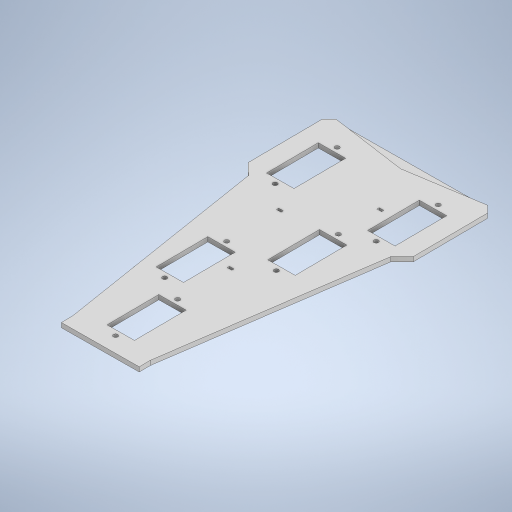
# Autodesk Inventor part: RevisedServoTray
Saved by Autodesk Inventor 2023 (Build 270158000, 158)
## iProperties
Created: 2023-05-02
Part Number: RevisedServoTray
Material: Generic
Document SubType Name: Modeling
Designer: 1roweste
Density: 1 g/cm^3
Appearance: Default
Author: 1roweste
Autodesk Inventor part; units mm, degrees
ref_plane "YZ Plane" through (0, 0, 0) normal (1, 0, 0) x (0, 1, 0)
ref_plane "XZ Plane" through (0, 0, 0) normal (0, 1, 0) x (-1, 0, 0)
ref_plane "Work Plane1" through (0, 2, 0) normal (0, 1, 0) x (1, 0, 0)
sketch "Sketch4" plane through (0, 2, 0) normal (0, 1, 0) x (1, 0, 0)
  line L0 (-81.9697, 60.7) -> (-81.9697, 62.7) projected
  line L1 (-81.9697, 62.7) -> (-80.9697, 62.7) projected
  line L2 (-80.9697, 62.7) -> (-80.9697, 60.7) projected
  line L3 (-80.9697, 60.7) -> (-81.9697, 60.7) projected
  line L4 (-81.9697, 49.6253) -> (-81.9697, 51.6253) projected
  line L5 (-81.9697, 51.6253) -> (-80.9697, 51.6253) projected
  line L6 (-80.9697, 51.6253) -> (-80.9697, 49.6253) projected
  line L7 (-80.9697, 49.6253) -> (-81.9697, 49.6253) projected
  line L8 (-81.9697, 71.7747) -> (-81.9697, 73.7747) projected
  line L9 (-81.9697, 73.7747) -> (-80.9697, 73.7747) projected
  line L10 (-80.9697, 73.7747) -> (-80.9697, 71.7747) projected
  line L11 (-80.9697, 71.7747) -> (-81.9697, 71.7747) projected
  line L12 (-81.9697, 38.5507) -> (-81.9697, 40.5507) projected
  line L13 (-81.9697, 40.5507) -> (-80.9697, 40.5507) projected
  line L14 (-80.9697, 40.5507) -> (-80.9697, 38.5507) projected
  line L15 (-80.9697, 38.5507) -> (-81.9697, 38.5507) projected
  line L16 (-81.9697, 82.8493) -> (-81.9697, 84.8493) projected
  line L17 (-81.9697, 84.8493) -> (-80.9697, 84.8493) projected
  line L18 (-80.9697, 84.8493) -> (-80.9697, 82.8493) projected
  line L19 (-80.9697, 82.8493) -> (-81.9697, 82.8493) projected
  line L20 (-61.9934, 117.9) -> (-84.9697, 94.9237) projected
  line L21 (-84.9697, 94.9237) -> (-89.9697, 61.7) projected
  line L22 (-89.9697, 61.7) -> (-84.9697, 28.4763) projected
  line L23 (-84.9697, 28.4763) -> (-61.9934, 5.5) projected
  line L24 (-61.9934, 5.5) -> (0, 5.5) projected
  line L25 (0, 5.5) -> (0, 117.9) projected
  line L26 (0, 117.9) -> (-61.9934, 117.9) projected
  line L27 (-89.9697, 61.7) -> (-84.9697, 94.9237) projected
  line L28 (-84.9697, 94.9237) -> (-220.5912, 94.9237)
  line L29 (-220.5912, 94.9237) -> (-220.5912, 28.4763)
  line L30 (-220.5912, 28.4763) -> (-84.9697, 28.4763)
  line L31 (-84.9697, 28.4763) -> (-84.9697, 94.9237)
  line L32 (-91.9697, 94.9237) -> (-91.9697, 28.4763)
  line L33 (-81.9697, 25.4763) -> (-223.5912, 25.4763)
  line L34 (-223.5912, 25.4763) -> (-223.5912, 97.9237)
  line L35 (-223.5912, 97.9237) -> (-81.9697, 97.9237)
  line L36 (-81.9697, 97.9237) -> (-81.9697, 25.4763)
  line L37 (-84.9697, 94.9237) -> (-84.9697, 28.4763) projected
  line L38 (-84.9697, 28.4763) -> (-87.9697, 25.4763)
  line L39 (-84.9697, 28.4763) -> (-80.7271, 28.4763) construction
  line L40 (-84.9697, 94.9237) -> (-87.9697, 97.9237)
  line L41 (-84.9697, 94.9237) -> (-80.7271, 94.9237) construction
  line L42 (-81.9697, 83.8493) -> (-220.5912, 83.8493)
  line L43 (-81.9697, 83.8493) -> (56.6518, 83.8493) construction
  line L44 (-81.9697, 72.7743) -> (-220.5912, 72.7743)
  line L45 (-81.9697, 61.6993) -> (-220.5912, 61.6993)
  line L46 (-81.9697, 50.6243) -> (-220.5912, 50.6243)
  line L47 (-81.9697, 39.5493) -> (-220.5912, 39.5493)
  circle A0 centre (-109.4697, 83.8493) radius 17.5
  circle A1 centre (-109.4697, 39.5493) radius 17.5
  circle A2 centre (-203.0912, 61.6993) radius 17.5
  line L48 (-182.3896, 71.2657) -> (-182.3896, 65.7743)
  line L49 (-182.3896, 65.7743) -> (-157.3896, 65.7743)
  line L50 (-157.3896, 65.7743) -> (-157.3896, 71.2657)
  arc A3 (-157.3896, 71.2657) -> (-157.3896, 74.283) centre (-156.0766, 72.7743) ccw
  line L51 (-157.3896, 74.283) -> (-157.3896, 79.7743)
  line L52 (-157.3896, 79.7743) -> (-182.3896, 79.7743)
  line L53 (-182.3896, 79.7743) -> (-182.3896, 74.283)
  arc A4 (-182.3896, 74.283) -> (-182.3896, 71.2657) centre (-183.7026, 72.7743) ccw
  line L54 (-181.3896, 66.7743) -> (-181.3896, 78.7743)
  line L55 (-181.3896, 78.7743) -> (-158.3896, 78.7743)
  line L56 (-158.3896, 78.7743) -> (-158.3896, 66.7743)
  line L57 (-158.3896, 66.7743) -> (-181.3896, 66.7743)
  circle A5 centre (-156.0766, 72.7743) radius 1
  circle A6 centre (-183.7026, 72.7743) radius 1
  line L58 (-169.8896, 78.7743) -> (-169.8896, 66.7743)
  line L59 (-158.3896, 72.7743) -> (-181.3896, 72.7743)
  circle A7 centre (-169.8896, 72.7743) radius 0.5
  line L60 (-121.9697, 82.3407) -> (-121.9697, 76.8493)
  line L61 (-121.9697, 76.8493) -> (-96.9697, 76.8493)
  line L62 (-96.9697, 76.8493) -> (-96.9697, 82.3407)
  arc A8 (-96.9697, 82.3407) -> (-96.9697, 85.358) centre (-95.6567, 83.8493) ccw
  line L63 (-96.9697, 85.358) -> (-96.9697, 90.8493)
  line L64 (-96.9697, 90.8493) -> (-121.9697, 90.8493)
  line L65 (-121.9697, 90.8493) -> (-121.9697, 85.358)
  arc A9 (-121.9697, 85.358) -> (-121.9697, 82.3407) centre (-123.2827, 83.8493) ccw
  line L66 (-120.9697, 77.8493) -> (-120.9697, 89.8493)
  line L67 (-120.9697, 89.8493) -> (-97.9697, 89.8493)
  line L68 (-97.9697, 89.8493) -> (-97.9697, 77.8493)
  line L69 (-97.9697, 77.8493) -> (-120.9697, 77.8493)
  circle A10 centre (-95.6567, 83.8493) radius 1
  circle A11 centre (-123.2827, 83.8493) radius 1
  line L70 (-109.4697, 89.8493) -> (-109.4697, 77.8493)
  line L71 (-97.9697, 83.8493) -> (-120.9697, 83.8493)
  circle A12 centre (-109.4697, 83.8493) radius 0.5
  line L72 (-155.1713, 49.1157) -> (-155.1713, 43.6243)
  line L73 (-155.1713, 43.6243) -> (-130.1713, 43.6243)
  line L74 (-130.1713, 43.6243) -> (-130.1713, 49.1157)
  arc A13 (-130.1713, 49.1157) -> (-130.1713, 52.133) centre (-128.8583, 50.6243) ccw
  line L75 (-130.1713, 52.133) -> (-130.1713, 57.6243)
  line L76 (-130.1713, 57.6243) -> (-155.1713, 57.6243)
  line L77 (-155.1713, 57.6243) -> (-155.1713, 52.133)
  arc A14 (-155.1713, 52.133) -> (-155.1713, 49.1157) centre (-156.4843, 50.6243) ccw
  line L78 (-154.1713, 44.6243) -> (-154.1713, 56.6243)
  line L79 (-154.1713, 56.6243) -> (-131.1713, 56.6243)
  line L80 (-131.1713, 56.6243) -> (-131.1713, 44.6243)
  line L81 (-131.1713, 44.6243) -> (-154.1713, 44.6243)
  circle A15 centre (-128.8583, 50.6243) radius 1
  circle A16 centre (-156.4843, 50.6243) radius 1
  line L82 (-142.6713, 56.6243) -> (-142.6713, 44.6243)
  line L83 (-131.1713, 50.6243) -> (-154.1713, 50.6243)
  circle A17 centre (-142.6713, 50.6243) radius 0.5
  circle A18 centre (-216.7852, 61.6993) radius 1
  arc A19 (-215.4722, 63.208) -> (-215.4722, 60.1907) centre (-216.7852, 61.6993) ccw
  circle A20 centre (-189.1592, 61.6993) radius 1
  arc A21 (-190.4722, 60.1907) -> (-190.4722, 63.208) centre (-189.1592, 61.6993) ccw
  line L84 (-215.4722, 54.6993) -> (-190.4722, 54.6993)
  line L85 (-191.4722, 55.6993) -> (-214.4722, 55.6993)
  circle A22 centre (-202.9722, 61.6993) radius 0.5
  line L86 (-191.4722, 67.6993) -> (-191.4722, 55.6993)
  line L87 (-190.4722, 63.208) -> (-190.4722, 68.6993)
  line L88 (-215.4722, 60.1907) -> (-215.4722, 54.6993)
  line L89 (-191.4722, 61.6993) -> (-214.4722, 61.6993)
  line L90 (-202.9722, 67.6993) -> (-202.9722, 55.6993)
  line L91 (-214.4722, 55.6993) -> (-214.4722, 67.6993)
  line L92 (-214.4722, 67.6993) -> (-191.4722, 67.6993)
  line L93 (-215.4722, 68.6993) -> (-215.4722, 63.208)
  line L94 (-190.4722, 68.6993) -> (-215.4722, 68.6993)
  line L95 (-190.4722, 54.6993) -> (-190.4722, 60.1907)
  line L96 (-96.9697, 32.5493) -> (-96.9697, 38.0407)
  circle A23 centre (-95.6567, 39.5493) radius 1
  line L97 (-97.9697, 45.5493) -> (-97.9697, 33.5493)
  line L98 (-96.9697, 41.058) -> (-96.9697, 46.5493)
  arc A24 (-96.9697, 38.0407) -> (-96.9697, 41.058) centre (-95.6567, 39.5493) ccw
  circle A25 centre (-123.2827, 39.5493) radius 1
  line L99 (-109.4697, 45.5493) -> (-109.4697, 33.5493)
  circle A26 centre (-109.4697, 39.5493) radius 0.5
  line L100 (-97.9697, 39.5493) -> (-120.9697, 39.5493)
  line L101 (-97.9697, 33.5493) -> (-120.9697, 33.5493)
  line L102 (-120.9697, 45.5493) -> (-97.9697, 45.5493)
  line L103 (-121.9697, 32.5493) -> (-96.9697, 32.5493)
  line L104 (-96.9697, 46.5493) -> (-121.9697, 46.5493)
  line L105 (-121.9697, 38.0407) -> (-121.9697, 32.5493)
  line L106 (-120.9697, 33.5493) -> (-120.9697, 45.5493)
  arc A27 (-121.9697, 41.058) -> (-121.9697, 38.0407) centre (-123.2827, 39.5493) ccw
  line L107 (-121.9697, 46.5493) -> (-121.9697, 41.058)
  circle A28 centre (-142.6713, 50.6243) radius 17.5
  circle A29 centre (-169.8896, 72.7743) radius 17.5
  point P0 (0, 0)
  point P1 (-154.188, 74.9293)
  dimension "d22" = 7
  dimension "d23" = 3
  dimension "d24" = 135
  dimension "d25" = 135
  dimension "d26" = 180
  dimension "d29" = 11.075
  dimension "d34" = 35
  dimension "d35" = 17.5
  dimension "d36" = 0
  dimension "d37" = 35
  dimension "d38" = 0
  dimension "d39" = 17.5
  dimension "d44" = 35
  dimension "d45" = 0
  dimension "d46" = 17.5
  dimension "d47" = 1
  dimension "d48" = 1
  dimension "d49" = 1
  dimension "d50" = 1
  dimension "d51" = 1
  dimension "d56" = 35
  dimension "d57" = 35
  constraints: 158 end point, 30 centre point, 25 midpoint, 20 point on circle, 8 point on line, 4 horizontal, 4 parallel, 3 equal length, 3 perpendicular, 2 equal radius, 1 vertical, 15 other
  measures "d22" distance between parallel lines of L31 L32
  measures "d23" distance between parallel lines of L30 L33
  measures "d24" angle of L38 L39
  measures "d25" angle of L41 L40
  measures "d26" angle of L42 L43
  measures "d29" distance of L42.start L44.start
  measures "d34" diameter of A0
  measures "d35" distance from line of L32 A0.centre
  measures "d36" distance from line of L42 A0.centre
  measures "d37" diameter of A1
  measures "d38" distance from line of L47 A1.centre
  measures "d39" distance from line of L32 A1.centre
  measures "d44" diameter of A2
  measures "d45" distance from line of L45 A2.centre
  measures "d46" distance from line of A2.centre L29
  measures "d47" diameter of A7
  measures "d48" diameter of A12
  measures "d49" diameter of A17
  measures "d50" diameter of A22
  measures "d51" diameter of A26
  measures "d56" diameter of A28
  measures "d57" diameter of A29
extrude "Extrusion4" add sketch "Sketch4" along normal blind 2 contours L45 L32 L44 L21 | L22 L46 L32 L45 | L22 L47 L32 L46 | L44 L32 L42 L21 | L45 A28 A29 L44 A0 L32 | L32 L46 A1 A28 L45 | L30 L32 L47 L22 | L38 L33 A1 L30 | L32 A1 L46 | L21 L42 L32 L28 | L28 A0 L35 L40 | L44 A0 L32 | A28 L46 A13 L75 L76 L77 A14 L45 | L45 A28 | L30 A1 L32 | A1 L30 L47 A27 L105 L103 L96 A24 | L47 A24 L98 L104 L107 A27 A1 L46 | L46 A1 | L32 A0 L28 | A0 L44 L42 A9 L60 L61 L62 A8 | L42 A8 L63 L64 L65 A9 A0 L28 | A0 L44 | A28 L46 A2 L45 A29 | A28 L47 L46 A14 L72 L73 L74 A13 | L46 A1 A28 | A1 L33 L30 | A24 L96 L103 L105 A27 L47 A25 L106 L101 L97 A23 | L47 A23 L97 L102 L106 A25 A27 L107 L104 L98 A24 | L28 A0 L35 | A8 L62 L61 L60 A9 L42 A11 L66 L69 L68 A10 | L42 A10 L68 L67 L66 A11 A9 L65 L64 L63 A8 | L44 A29 L42 A0 | A29 L45 | L45 A29 L44 A4 L48 L49 L50 A3 | A28 L47 L29 L46 A2 | A13 L74 L73 L72 A14 L46 A16 L78 L81 L80 A15 | L46 A15 L80 L79 L78 A16 A14 L77 L76 L75 A13 | A1 L47 A28 | A1 L33 L34 L35 A0 L28 L29 L30 | L30 L29 L47 A28 A1 | A0 L42 A29 L29 L28 | L44 A3 L51 L52 L53 A4 A29 L42 | L45 A2 A29 | A2 L46 | L46 A2 L45 A19 L88 L84 L95 A21 | L47 A28 | A3 L50 L49 L48 A4 L44 A6 L54 L57 L56 A5 | L44 A5 L56 L55 L54 A6 A4 L53 L52 L51 A3 | L42 A29 | L45 A21 L87 L94 L93 A19 A2 L44 | A2 L44 A29 | L46 L29 A2 | L42 A29 L44 A2 L29 | A21 L95 L84 L88 A19 L45 A18 L91 L85 L86 A20 | L45 A20 L86 L92 L91 A18 A19 L93 L94 L87 A21 | L44 A2 | L29 L44 A2
extrude "Extrusion5" add sketch "Sketch4" along normal blind 1 contours L45 L21 L44 L31 | L31 L46 L22 L45 | L31 L47 L22 L46 | L44 L21 L42 L31 | L31 L22 L47 | L42 L21 L31
sketch "Sketch5" plane through (0, 2, 0) normal (0, -1, 0) x (1, 0, 0)
  line L0 (-131.8896, -71.7743) -> (-132.8896, -71.7743)
  line L1 (-132.8896, -71.7743) -> (-132.8896, -73.7743)
  line L2 (-132.8896, -73.7743) -> (-131.8896, -73.7743)
  line L3 (-131.8896, -73.7743) -> (-131.8896, -71.7743)
  line L4 (-81.9697, -50.6243) -> (-220.5912, -50.6243) projected
  line L5 (-81.9697, -61.6993) -> (-220.5912, -61.6993) projected
  line L6 (-81.9697, -72.7743) -> (-220.5912, -72.7743) projected
  circle A0 centre (-169.8896, -72.7743) radius 17.5 projected
  circle A1 centre (-203.0912, -61.6993) radius 17.5 projected
  circle A2 centre (-142.6713, -50.6243) radius 17.5 projected
  line L7 (-109.6713, -49.6243) -> (-110.6713, -49.6243)
  line L8 (-110.6713, -49.6243) -> (-110.6713, -51.6243)
  line L9 (-110.6713, -51.6243) -> (-109.6713, -51.6243)
  line L10 (-109.6713, -51.6243) -> (-109.6713, -49.6243)
  line L11 (-165.0912, -60.6993) -> (-166.0912, -60.6993)
  line L12 (-166.0912, -60.6993) -> (-166.0912, -62.6993)
  line L13 (-166.0912, -62.6993) -> (-165.0912, -62.6993)
  line L14 (-165.0912, -62.6993) -> (-165.0912, -60.6993)
  point P0 (0, 0)
  point P1 (-132.8896, -72.7743)
  point P2 (-132.3896, -73.7743)
  point P3 (-110.6713, -50.6243)
  point P4 (-110.1713, -51.6243)
  point P5 (-166.0912, -61.6993)
  point P6 (-165.5912, -60.6993)
  dimension "d58" = 1
  dimension "d59" = 2
  dimension "d60" = 0
  dimension "d61" = 37.5
  dimension "d62" = 1
  dimension "d63" = 2
  dimension "d64" = 0
  dimension "d65" = 32.5
  dimension "d66" = 1
  dimension "d67" = 2
  dimension "d68" = 0
  dimension "d69" = 37.5
  constraints: 24 end point, 6 midpoint, 6 parallel, 3 horizontal, 3 perpendicular, 1 horizontal alignment
  measures "d58" distance of L2.end L1.end
  measures "d59" distance of L1.end L0.end
  measures "d60" distance from line of L6 point (-132.89, -72.774)
  measures "d61" horizontal distance of A0.centre point (-132.39, -73.774)
  measures "d62" distance of L9.end L8.end
  measures "d63" distance of L8.end L7.end
  measures "d64" distance from line of L4 point (-110.671, -50.624)
  measures "d65" horizontal distance of A2.centre point (-110.171, -51.624)
  measures "d66" distance of L13.end L12.end
  measures "d67" distance of L12.end L11.end
  measures "d68" distance from line of L5 point (-166.091, -61.699)
  measures "d69" horizontal distance of point (-203.091, -61.699) point (-165.591, -60.699)
extrude "Extrusion6" cut sketch "Sketch5" against normal up to surface (2 mm away) contours L3 L6 L1 L0 | L8 L7 L10 L4 | L4 L10 L9 L8 | L3 L2 L1 L6 | L14 L13 L12 L5 | L5 L12 L11 L14
sketch "Sketch6" plane through (0, 4, 0) normal (0, 1, 0) x (1, 0, 0)
  line L0 (-166.0912, 62.6993) -> (-165.0912, 62.6993) projected
  line L1 (-165.0912, 62.6993) -> (-165.0912, 60.6993) projected
  line L2 (-165.0912, 60.6993) -> (-166.0912, 60.6993) projected
  line L3 (-166.0912, 60.6993) -> (-166.0912, 62.6993) projected
  line L4 (-110.6713, 51.6243) -> (-109.6713, 51.6243) projected
  line L5 (-109.6713, 51.6243) -> (-109.6713, 49.6243) projected
  line L6 (-109.6713, 49.6243) -> (-110.6713, 49.6243) projected
  line L7 (-110.6713, 49.6243) -> (-110.6713, 51.6243) projected
  line L8 (-131.8896, 73.7743) -> (-131.8896, 71.7743) projected
  line L9 (-131.8896, 71.7743) -> (-132.8896, 71.7743) projected
  line L10 (-132.8896, 71.7743) -> (-132.8896, 73.7743) projected
  line L11 (-132.8896, 73.7743) -> (-131.8896, 73.7743) projected
  line L12 (-84.9697, 94.9237) -> (-87.9697, 97.9237) projected
  line L13 (-87.9697, 97.9237) -> (-223.5912, 97.9237) projected
  line L14 (-223.5912, 97.9237) -> (-223.5912, 25.4763) projected
  line L15 (-223.5912, 25.4763) -> (-87.9697, 25.4763) projected
  line L16 (-87.9697, 25.4763) -> (-84.9697, 28.4763) projected
  line L17 (-84.9697, 28.4763) -> (-89.9697, 61.7) projected
  line L18 (-89.9697, 61.7) -> (-84.9697, 94.9237) projected
  line L19 (-181.3896, 66.7743) -> (-181.3896, 78.7743) projected
  line L20 (-181.3896, 78.7743) -> (-158.3896, 78.7743) projected
  line L21 (-158.3896, 78.7743) -> (-158.3896, 66.7743) projected
  line L22 (-158.3896, 66.7743) -> (-181.3896, 66.7743) projected
  circle A0 centre (-156.0766, 72.7743) radius 1 projected
  line L23 (-120.9697, 77.8493) -> (-120.9697, 89.8493) projected
  line L24 (-120.9697, 89.8493) -> (-97.9697, 89.8493) projected
  line L25 (-97.9697, 89.8493) -> (-97.9697, 77.8493) projected
  line L26 (-97.9697, 77.8493) -> (-120.9697, 77.8493) projected
  circle A1 centre (-95.6567, 83.8493) radius 1 projected
  circle A2 centre (-156.4843, 50.6243) radius 1 projected
  line L27 (-154.1713, 44.6243) -> (-154.1713, 56.6243) projected
  line L28 (-154.1713, 56.6243) -> (-131.1713, 56.6243) projected
  line L29 (-131.1713, 56.6243) -> (-131.1713, 44.6243) projected
  line L30 (-131.1713, 44.6243) -> (-154.1713, 44.6243) projected
  circle A3 centre (-216.7852, 61.6993) radius 1 projected
  line L31 (-214.4722, 55.6993) -> (-214.4722, 67.6993) projected
  line L32 (-214.4722, 67.6993) -> (-191.4722, 67.6993) projected
  line L33 (-191.4722, 67.6993) -> (-191.4722, 55.6993) projected
  line L34 (-191.4722, 55.6993) -> (-214.4722, 55.6993) projected
  circle A4 centre (-123.2827, 39.5493) radius 1 projected
  line L35 (-120.9697, 33.5493) -> (-120.9697, 45.5493) projected
  line L36 (-120.9697, 45.5493) -> (-97.9697, 45.5493) projected
  line L37 (-97.9697, 45.5493) -> (-97.9697, 33.5493) projected
  line L38 (-97.9697, 33.5493) -> (-120.9697, 33.5493) projected
  circle A5 centre (-95.6567, 39.5493) radius 1 projected
  circle A6 centre (-189.1592, 61.6993) radius 1 projected
  circle A7 centre (-183.7026, 72.7743) radius 1 projected
  circle A8 centre (-123.2827, 83.8493) radius 1 projected
  circle A9 centre (-128.8583, 50.6243) radius 1 projected
  line L39 (-153.3896, 83.7743) -> (-186.3896, 83.7743)
  line L40 (-186.3896, 83.7743) -> (-186.3896, 61.7743)
  line L41 (-186.3896, 61.7743) -> (-153.3896, 61.7743)
  line L42 (-153.3896, 61.7743) -> (-153.3896, 83.7743)
  line L43 (-218.5912, 92.9237) -> (-90.327, 92.9237)
  line L44 (-90.327, 92.9237) -> (-95.026, 61.7)
  line L45 (-95.026, 61.7) -> (-90.327, 30.4763)
  line L46 (-90.327, 30.4763) -> (-218.5912, 30.4763)
  line L47 (-218.5912, 30.4763) -> (-218.5912, 92.9237)
  line L48 (-125.9697, 94.8493) -> (-125.9697, 72.8493)
  line L49 (-125.9697, 72.8493) -> (-92.9697, 72.8493)
  line L50 (-92.9697, 72.8493) -> (-92.9697, 94.8493)
  line L51 (-92.9697, 94.8493) -> (-125.9697, 94.8493)
  line L52 (-125.9697, 50.5493) -> (-125.9697, 28.5493)
  line L53 (-125.9697, 28.5493) -> (-92.9697, 28.5493)
  line L54 (-92.9697, 28.5493) -> (-92.9697, 50.5493)
  line L55 (-92.9697, 50.5493) -> (-125.9697, 50.5493)
  line L56 (-186.4722, 72.6993) -> (-219.4722, 72.6993)
  line L57 (-219.4722, 72.6993) -> (-219.4722, 50.6993)
  line L58 (-219.4722, 50.6993) -> (-186.4722, 50.6993)
  line L59 (-186.4722, 50.6993) -> (-186.4722, 72.6993)
  line L60 (-125.9697, 92.9237) -> (-218.5912, 78.7743)
  line L61 (-125.9697, 30.4763) -> (-218.5912, 44.6243)
  line L62 (-125.9697, 92.9237) -> (-120.9697, 97.9237)
  line L63 (-125.9697, 30.4763) -> (-120.9697, 25.4763)
  line L64 (-223.5912, 25.4763) -> (-87.9697, 25.4763) projected
  line L65 (-218.5912, 78.7743) -> (-223.5912, 78.7743)
  line L66 (-218.5912, 44.6243) -> (-223.5912, 44.6243)
  point P0 (0, 0)
  point P1 (-186.3896, 83.6936)
  point P2 (-185.8613, 83.7743)
  dimension "d72" = 5
  dimension "d73" = 5
  dimension "d74" = 5
  dimension "d75" = 5
  dimension "d76" = 5
  constraints: 54 end point, 10 point on line, 2 perpendicular, 16 other
  measures "d72" distance between parallel lines of L20 L39
  measures "d73" distance between parallel lines of L13 L43
  measures "d74" distance between parallel lines of L23 L48
  measures "d75" distance between parallel lines of L35 L52
  measures "d76" distance between parallel lines of L32 L56
extrude "Extrusion7" cut sketch "Sketch6" against normal blind 10 contours L60 L47 L43 L39 L40 | L65 L14 L13 L62 L51 L48 L43 L47 | L48 L51 L62 | L66 L47 L46 L52 L53 L63 L15 L14 | L61 L46 L47 | L63 L53 L52
body "Solid2"
